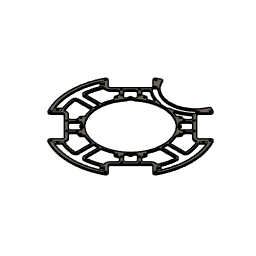
Frame_underside v16 (Autodesk Fusion 360 design; units mm, degrees)
Autodesk Fusion 360 part; units mm, degrees
note: some values were not read from the file. Set by a fixed rule: which face or edge a step refers to.
(part 1 of 3)
sketch "スケッチ1" plane through (0, 0, 0) normal (0, 0, 1) x (1, 0, 0)
  circle A0 centre (0, 0) radius 108
  circle A1 centre (0, 115.48) radius 45
  line L0 (0, 0) -> (76.3675, 76.3675)
  line L1 (0, 0) -> (108, 0) construction
  line L2 (0, 0) -> (76.3675, -76.3675)
  line L3 (76.3675, 76.3675) -> (58.5484, 58.5484)
  line L4 (76.3675, 76.3675) -> (96.1665, 56.5685)
  line L5 (76.3675, 76.3675) -> (56.5685, 96.1665)
  line L6 (96.1665, 56.5685) -> (78.3474, 38.7495)
  line L7 (78.3474, 38.7495) -> (58.5484, 58.5484)
  line L8 (56.5685, 96.1665) -> (38.7495, 78.3474)
  line L9 (38.7495, 78.3474) -> (58.5484, 58.5484)
  line L10 (56.5685, -96.1665) -> (38.7495, -78.3474)
  line L11 (38.7495, -78.3474) -> (58.5484, -58.5484)
  line L12 (78.3474, -38.7495) -> (58.5484, -58.5484)
  line L13 (96.1665, -56.5685) -> (78.3474, -38.7495)
  line L14 (76.3675, -76.3675) -> (96.1665, -56.5685)
  line L15 (76.3675, -76.3675) -> (56.5685, -96.1665)
  line L16 (0, 2.5) -> (0, 20)
  line L17 (-56.5685, -96.1665) -> (-38.7495, -78.3474)
  line L18 (-38.7495, -78.3474) -> (-58.5484, -58.5484)
  line L19 (-78.3474, -38.7495) -> (-58.5484, -58.5484)
  line L20 (-96.1665, -56.5685) -> (-78.3474, -38.7495)
  line L21 (-76.3675, -76.3675) -> (-96.1665, -56.5685)
  line L22 (-76.3675, -76.3675) -> (-56.5685, -96.1665)
  line L23 (0, 0) -> (-76.3675, -76.3675)
  line L24 (0, 0) -> (-76.3675, 76.3675)
  line L25 (-38.7495, 78.3474) -> (-58.5484, 58.5484)
  line L26 (-78.3474, 38.7495) -> (-58.5484, 58.5484)
  line L27 (-56.5685, 96.1665) -> (-38.7495, 78.3474)
  line L28 (-76.3675, 76.3675) -> (-56.5685, 96.1665)
  line L29 (-76.3675, 76.3675) -> (-96.1665, 56.5685)
  line L30 (-96.1665, 56.5685) -> (-78.3474, 38.7495)
  line L31 (-96.1665, 56.5685) -> (-99.7021, 53.033)
  line L32 (-99.7021, 53.033) -> (-78.3474, 31.6784)
  line L33 (-78.3474, 31.6784) -> (-31.6784, 78.3474)
  line L34 (-31.6784, 78.3474) -> (-53.033, 99.7021)
  line L35 (-53.033, 99.7021) -> (-56.5685, 96.1665)
  line L36 (-99.7021, -53.033) -> (-78.3474, -31.6784)
  line L37 (-78.3474, -31.6784) -> (-31.6784, -78.3474)
  line L38 (-31.6784, -78.3474) -> (-53.033, -99.7021)
  line L39 (-96.1665, -56.5685) -> (-99.7021, -53.033)
  line L40 (-53.033, -99.7021) -> (-56.5685, -96.1665)
  line L41 (96.1665, -56.5685) -> (99.7021, -53.033)
  line L42 (99.7021, -53.033) -> (78.3474, -31.6784)
  line L43 (78.3474, -31.6784) -> (31.6784, -78.3474)
  line L44 (31.6784, -78.3474) -> (53.033, -99.7021)
  line L45 (53.033, -99.7021) -> (56.5685, -96.1665)
  line L46 (96.1665, 56.5685) -> (99.7021, 53.033)
  line L47 (99.7021, 53.033) -> (78.3474, 31.6784)
  line L48 (78.3474, 31.6784) -> (31.6784, 78.3474)
  line L49 (31.6784, 78.3474) -> (53.033, 99.7021)
  line L50 (53.033, 99.7021) -> (56.5685, 96.1665)
  line L51 (-108, 0) -> (-103, 0)
  circle A2 centre (0, 0) radius 103
  line L52 (-103, 0) -> (-93, 0)
  circle A3 centre (0, 0) radius 93
  line L53 (0, 115.48) -> (0, 70.48)
  line L54 (0, 70.48) -> (0, 68.48)
  line L55 (0, 68.48) -> (0, 60.48)
  circle A4 centre (0, 115.48) radius 47
  circle A5 centre (0, 115.48) radius 55
  line L56 (0, 60.48) -> (0, 58.48)
  circle A6 centre (0, 115.48) radius 57
  line L57 (-93, 0) -> (-90, 0)
  circle A7 centre (0, 0) radius 90
  line L58 (0, 60.48) -> (0, 57.48)
  circle A8 centre (0, 0) radius 57.48
  circle A9 centre (0, 0) radius 60.48
  circle A10 centre (-42.7658, 42.7658) radius 3
  circle A11 centre (-42.7658, 42.7658) radius 1.45
  line L59 (-42.7658, 42.7658) -> (-44.8871, 40.6445)
  line L60 (-44.8871, 40.6445) -> (-42.1834, 37.9407)
  line L61 (-42.1834, 37.9407) -> (-37.9407, 42.1834)
  line L62 (-37.9407, 42.1834) -> (-42.7658, 42.7658)
  line L63 (-42.7658, 42.7658) -> (-40.6445, 44.8871)
  line L64 (-40.6445, 44.8871) -> (-37.9407, 42.1834)
  circle A12 centre (-42.7658, -42.7658) radius 3
  circle A13 centre (-42.7658, -42.7658) radius 1.45
  line L65 (-40.6445, -44.8871) -> (-37.9407, -42.1834)
  line L66 (-37.9407, -42.1834) -> (-42.1834, -37.9407)
  line L67 (-44.8871, -40.6445) -> (-42.1834, -37.9407)
  line L68 (-42.7658, -42.7658) -> (-44.8871, -40.6445)
  line L69 (-42.7658, -42.7658) -> (-40.6445, -44.8871)
  circle A14 centre (42.7658, -42.7658) radius 3
  circle A15 centre (42.7658, -42.7658) radius 1.45
  line L70 (44.8871, -40.6445) -> (42.1834, -37.9407)
  line L71 (42.1834, -37.9407) -> (37.9407, -42.1834)
  line L72 (40.6445, -44.8871) -> (37.9407, -42.1834)
  line L73 (42.7658, -42.7658) -> (40.6445, -44.8871)
  line L74 (42.7658, -42.7658) -> (44.8871, -40.6445)
  circle A16 centre (42.7658, 42.7658) radius 3
  circle A17 centre (42.7658, 42.7658) radius 1.45
  line L75 (40.6445, 44.8871) -> (37.9407, 42.1834)
  line L76 (37.9407, 42.1834) -> (42.1834, 37.9407)
  line L77 (44.8871, 40.6445) -> (42.1834, 37.9407)
  line L78 (42.7658, 42.7658) -> (44.8871, 40.6445)
  line L79 (42.7658, 42.7658) -> (40.6445, 44.8871)
  line L80 (-103, 0) -> (-103, 5)
  line L81 (-103, 5) -> (-57.2621, 5)
  line L82 (-103, 0) -> (-103, -5)
  line L83 (-103, -5) -> (-57.2621, -5)
  line L84 (-103, 5) -> (-103, 8)
  line L85 (-103, 8) -> (-56.9206, 8)
  line L86 (-103, -5) -> (-103, -8)
  line L87 (-103, -8) -> (-56.9206, -8)
  line L88 (103, 8) -> (56.9206, 8)
  line L89 (103, 5) -> (57.2621, 5)
  line L90 (103, -5) -> (57.2621, -5)
  line L91 (103, -8) -> (56.9206, -8)
  line L92 (0, -108) -> (5, -108)
  line L93 (5, -108) -> (0, -108)
  line L94 (0, -108) -> (0, -57.4798)
  line L95 (0, -57.4798) -> (5, -57.4798)
  line L96 (5, -57.4798) -> (5, -108)
  line L97 (0, -108) -> (-5, -108)
  line L98 (-5, -108) -> (-5, -57.4798)
  line L99 (-5, -57.4798) -> (0, -57.4798)
  line L100 (0, -57.4798) -> (0, -108)
  line L101 (-5, -57.4798) -> (-8, -57.4798)
  line L102 (-8, -57.4798) -> (-8, -108)
  line L103 (-8, -108) -> (-5, -108)
  line L104 (-5, -108) -> (-5, -57.4798)
  line L105 (5, -108) -> (8, -108)
  line L106 (8, -108) -> (8, -57.4798)
  line L107 (8, -57.4798) -> (5, -57.4798)
  line L108 (5, -57.4798) -> (5, -108)
  line L109 (0, -108) -> (0, -104.5)
  circle A18 centre (0, 0) radius 104.5
  line L110 (-31.6784, -78.3474) -> (-32.739, -77.2868)
  line L111 (-32.739, -77.2868) -> (-50.7732, -95.3209)
  circle A19 centre (-48.1818, -92.7295) radius 1.65
  line L112 (-78.3474, -31.6784) -> (-77.2868, -32.739)
  line L113 (-77.2868, -32.739) -> (-98.6414, -54.0937)
  circle A20 centre (-92.7295, -48.1818) radius 1.65
  line L114 (31.6784, -78.3474) -> (32.739, -77.2868)
  line L115 (32.739, -77.2868) -> (54.0937, -98.6414)
  circle A21 centre (48.1818, -92.7295) radius 1.65
  line L116 (78.3474, -31.6784) -> (77.2868, -32.739)
  line L117 (77.2868, -32.739) -> (98.6414, -54.0937)
  circle A22 centre (92.7295, -48.1818) radius 1.65
  line L118 (-99.7021, 53.033) -> (-98.6414, 54.0937)
  line L119 (-98.6414, 54.0937) -> (-77.2868, 32.739)
  circle A23 centre (-92.7295, 48.1818) radius 1.65
  circle A24 centre (92.7295, -48.1818) radius 1.65
  circle A25 centre (48.1818, 92.7295) radius 1.65
  circle A26 centre (-92.7295, 48.1818) radius 1.65
  line L120 (31.6784, 78.3474) -> (32.739, 77.2868)
  line L121 (32.739, 77.2868) -> (54.0937, 98.6414)
  circle A27 centre (48.1818, -92.7295) radius 1.65
  circle A28 centre (92.7295, 48.1818) radius 1.65
  circle A29 centre (-48.1818, 92.7295) radius 1.65
  line L122 (-58.5484, 58.5484) -> (-66.4857, 50.6112)
  line L123 (-66.4857, 50.6112) -> (-50.6112, 66.4857)
  line L124 (-50.6112, 66.4857) -> (-29.0444, 44.919)
  line L125 (-29.0444, 44.919) -> (-44.919, 29.0444)
  line L126 (-44.919, 29.0444) -> (-66.4857, 50.6112)
  line L127 (-66.4857, 50.6112) -> (-64.7179, 52.3789)
  line L128 (-64.7179, 52.3789) -> (-43.1512, 30.8122)
  line L129 (-66.4857, 50.6112) -> (-68.2535, 48.8434)
  line L130 (-68.2535, 48.8434) -> (-46.6867, 27.2766)
  line L131 (-46.6867, 27.2766) -> (-44.919, 29.0444)
  line L132 (-48.8434, 68.2535) -> (-27.2766, 46.6867)
  line L133 (-52.3789, 64.7179) -> (-30.8122, 43.1512)
  line L134 (-29.0444, 44.919) -> (-27.2766, 46.6867)
  line L135 (-66.4857, 50.6112) -> (-64.0816, 48.207)
  circle A30 centre (-64.0816, 48.207) radius 1.65
  circle A31 centre (-48.207, 64.0816) radius 1.65
  line L136 (-64.0816, 48.207) -> (-55.172, 39.2975)
  line L137 (-55.172, 39.2975) -> (-39.2975, 55.172)
  circle A32 centre (-55.172, 39.2975) radius 1.65
  circle A33 centre (-39.2975, 55.172) radius 1.65
  circle A34 centre (-48.207, -64.0816) radius 1.65
  circle A35 centre (-39.2975, -55.172) radius 1.65
  circle A36 centre (-64.0816, -48.207) radius 1.65
  circle A37 centre (-55.172, -39.2975) radius 1.65
  line L138 (-64.7179, -52.3789) -> (-43.1512, -30.8122)
  line L139 (-68.2535, -48.8434) -> (-46.6867, -27.2766)
  line L140 (-44.919, -29.0444) -> (-46.6867, -27.2766)
  line L141 (-27.2766, -46.6867) -> (-29.0444, -44.919)
  line L142 (-48.8434, -68.2535) -> (-27.2766, -46.6867)
  line L143 (-29.0444, -44.919) -> (-50.6112, -66.4857)
  line L144 (-52.3789, -64.7179) -> (-30.8122, -43.1512)
  line L145 (-44.919, -29.0444) -> (-29.0444, -44.919)
  line L146 (-66.4857, -50.6112) -> (-44.919, -29.0444)
  circle A38 centre (64.0816, -48.207) radius 1.65
  circle A39 centre (55.172, -39.2975) radius 1.65
  circle A40 centre (48.207, -64.0816) radius 1.65
  circle A41 centre (39.2975, -55.172) radius 1.65
  line L147 (52.3789, -64.7179) -> (30.8122, -43.1512)
  line L148 (48.8434, -68.2535) -> (27.2766, -46.6867)
  line L149 (29.0444, -44.919) -> (27.2766, -46.6867)
  line L150 (46.6867, -27.2766) -> (44.919, -29.0444)
  line L151 (68.2535, -48.8434) -> (46.6867, -27.2766)
  line L152 (44.919, -29.0444) -> (66.4857, -50.6112)
  line L153 (64.7179, -52.3789) -> (43.1512, -30.8122)
  line L154 (29.0444, -44.919) -> (44.919, -29.0444)
  line L155 (50.6112, -66.4857) -> (29.0444, -44.919)
  circle A42 centre (48.207, 64.0816) radius 1.65
  circle A43 centre (39.2975, 55.172) radius 1.65
  circle A44 centre (64.0816, 48.207) radius 1.65
  circle A45 centre (55.172, 39.2975) radius 1.65
  line L156 (64.7179, 52.3789) -> (43.1512, 30.8122)
  line L157 (68.2535, 48.8434) -> (46.6867, 27.2766)
  line L158 (44.919, 29.0444) -> (46.6867, 27.2766)
  line L159 (27.2766, 46.6867) -> (29.0444, 44.919)
  line L160 (48.8434, 68.2535) -> (27.2766, 46.6867)
  line L161 (29.0444, 44.919) -> (50.6112, 66.4857)
  line L162 (52.3789, 64.7179) -> (30.8122, 43.1512)
  line L163 (44.919, 29.0444) -> (29.0444, 44.919)
  line L164 (66.4857, 50.6112) -> (44.919, 29.0444)
  line L165 (-60.273, 5) -> (-60.273, -5)
  line L166 (-31.6784, 78.3474) -> (-28.9756, 81.0502)
  line L167 (31.6784, 78.3474) -> (28.9756, 81.0502)
  line L168 (60.273, -5) -> (60.273, 5)
  line L169 (-5, -60.273) -> (5, -60.273)
  line L170 (-38.7495, 78.3474) -> (-34.0326, 83.0643)
  line L171 (38.7495, 78.3474) -> (32.618, 84.4789)
  line L172 (38.7495, 78.3474) -> (38.0423, 77.6403)
  line L173 (38.0423, 77.6403) -> (31.921, 83.7617)
  line L174 (-38.7495, 78.3474) -> (-38.0423, 77.6403)
  line L175 (-38.0423, 77.6403) -> (-33.3352, 82.3475)
  line L176 (-38.0423, 77.6403) -> (-40.4063, 75.2764)
  line L177 (38.0423, 77.6403) -> (40.4063, 75.2764)
  dimension "d1" = 216
  dimension "d2" = 90
  dimension "d4" = 45
  dimension "d5" = 25.2
  dimension "d6" = 28
  dimension "d7" = 28
  dimension "d9" = 25.2
  dimension "d10" = 28
  dimension "d11" = 25.2
  dimension "d12" = 28
  dimension "d13" = 5
  dimension "d14" = 30.2
  dimension "d15" = 66
  dimension "d16" = 30.2
  dimension "d17" = 5
  dimension "d18" = 10
  dimension "d20" = 2
  dimension "d21" = 8
  dimension "d22" = 2
  dimension "d23" = 3
  dimension "d24" = 3
  dimension "d25" = 2.9
  dimension "d26" = 6
  dimension "d27" = 3
  dimension "d29" = 360
  dimension "d30" = 5
  dimension "d31" = 5
  dimension "d32" = 3
  dimension "d33" = 3
  dimension "d34" = 5
  dimension "d35" = 5
  dimension "d36" = 5
  dimension "d37" = 3
  dimension "d38" = 3
  dimension "d39" = 3.5
  dimension "d40" = 1.5
  dimension "d42" = 3.3
  dimension "d43" = 1.5
  dimension "d45" = 3.3
  dimension "d46" = 1.5
  dimension "d48" = 3.3
  dimension "d49" = 1.5
  dimension "d51" = 3.3
  dimension "d52" = 1.5
  dimension "d54" = 3.3
  dimension "d56" = 360
  dimension "d57" = 1.5
  dimension "d59" = 360
  dimension "d60" = 11.225
  dimension "d61" = 22.45
  dimension "d62" = 30.5
  dimension "d63" = 22.45
  dimension "d64" = 2.5
  dimension "d65" = 2.5
  dimension "d66" = 30.5
  dimension "d67" = 3.4
  dimension "d68" = 3.3
  dimension "d69" = 12.6
  dimension "d70" = 22.45
  dimension "d71" = 3.3
  dimension "d72" = 3.3
  dimension "d74" = 360
  dimension "d77" = 1
  constraint coincident A0.centre L0.start
  constraint horizontal L1
  constraint coincident A0 L0.end
  constraint coincident A0 L2.end
  constraint perpendicular L0 L2
  constraint perpendicular L2 L3
  constraint perpendicular L3 L4
  constraint perpendicular L0 L5
  constraint perpendicular L4 L6
  constraint perpendicular L6 L7
  constraint perpendicular L5 L8
  constraint perpendicular L8 L9
  constraint symmetric L0.end L1 L2.end
  constraint symmetric L1 L4.end L13.start
  constraint symmetric L1 L5.end L10.start
  constraint symmetric L1 L6.end L12.start
  constraint symmetric L1 L3.end L11.end
  constraint symmetric L1 L8.end L10.end
  constraint symmetric A0.centre L16 L0.start
  constraint symmetric L0.end L16 L24.end
  constraint symmetric L2.end L16 L21.start
  constraint symmetric L4.end L16 L29.end
  constraint symmetric L5.end L16 L27.start
  constraint symmetric L6.end L16 L26.start
  constraint symmetric L3.end L16 L25.end
  constraint symmetric L8.end L16 L25.start
  constraint symmetric L10.start L16 L17.start
  constraint symmetric L10.end L16 L17.end
  constraint symmetric L11.end L16 L18.end
  constraint symmetric L12.start L16 L19.start
  constraint symmetric L13.start L16 L20.start
  constraint perpendicular L30 L31
  constraint perpendicular L26 L32
  constraint perpendicular L32 L33
  constraint perpendicular L33 L34
  constraint symmetric L1 L27.start L17.start
  constraint symmetric L1 L29.end L20.start
  constraint symmetric L1 L31.end L36.start
  constraint symmetric L1 L32.end L36.end
  constraint symmetric L1 L33.end L37.end
  constraint symmetric L1 L34.end L38.end
  constraint symmetric L16 L27.start L5.end
  constraint symmetric L16 L29.end L4.end
  constraint symmetric L16 L31.end L46.end
  constraint symmetric L16 L32.end L47.end
  constraint symmetric L16 L33.end L48.end
  constraint symmetric L16 L34.end L49.end
  constraint symmetric L16 L36.start L41.end
  constraint symmetric L16 L36.end L42.end
  constraint symmetric L16 L37.end L43.end
  constraint symmetric L16 L38.end L44.end
  constraint symmetric L16 L20.start L13.start
  constraint symmetric L16 L17.start L10.start
  constraint coincident A0 L51.start
  constraint horizontal L51
  constraint coincident L51.end A2
  constraint parallel L51 L52
  constraint coincident L52.end A3
  constraint coincident A1.centre L53.start
  constraint coincident A1 L53.end
  constraint vertical L53
  constraint parallel L53 L54
  constraint parallel L53 L55
  constraint concentric A1 A4
  constraint coincident L54.end A4
  constraint concentric A1 A5
  constraint coincident L55.end A5
  constraint parallel L55 L56
  constraint concentric A4 A6
  constraint coincident L56.end A6
  constraint concentric A2 A7
  constraint coincident L57.end A7
  constraint parallel L56 L58
  constraint concentric A7 A8
  constraint coincident L58.end A8
  constraint concentric A3 A9
  constraint coincident L55.end A9
  constraint tangent A5 A9
  constraint coincident A9 A10.centre
  constraint coincident L24 A10.centre
  constraint tangent A8 A10
  constraint concentric A10 A11
  constraint coincident A10.centre A11.centre
  constraint coincident A10 L59.end
  constraint tangent A9 L59
  constraint perpendicular L24 L59
  constraint tangent A10 L60
  constraint perpendicular L24 L61
  constraint tangent A9 L63
  constraint perpendicular L52 L80
  constraint coincident A8 L81.end
  constraint perpendicular L80 L81
  constraint perpendicular L52 L82
  constraint coincident A8 L83.end
  constraint perpendicular L82 L83
  constraint perpendicular L81 L84
  constraint coincident A8 L85.end
  constraint perpendicular L84 L85
  constraint perpendicular L83 L86
  constraint coincident A8 L87.end
  constraint perpendicular L86 L87
  constraint symmetric L16 L80.end L89.start
  constraint symmetric L16 L81.end L89.end
  constraint symmetric L16 L82.end L90.start
  constraint symmetric L16 L83.end L90.end
  constraint symmetric L16 L84.end L88.start
  constraint symmetric L16 L85.end L88.end
  constraint symmetric L16 L86.end L91.start
  constraint symmetric L16 L87.end L91.end
  constraint coincident A0 L92.start
  constraint horizontal L92
  constraint horizontal L93
  constraint vertical L94
  constraint horizontal L95
  constraint vertical L96
  constraint horizontal L97
  constraint vertical L98
  constraint horizontal L99
  constraint vertical L100
  constraint horizontal L101
  constraint vertical L102
  constraint horizontal L103
  constraint vertical L104
  constraint horizontal L105
  constraint vertical L106
  constraint horizontal L107
  constraint vertical L108
  constraint perpendicular L97 L109
  constraint concentric A3 A18
  constraint coincident L109.end A18
  constraint coincident L37 L110.end
  constraint coincident A0 L111.end
  constraint perpendicular L110 L111
  constraint perpendicular L36 L112
  constraint coincident L39 L113.end
  constraint perpendicular L39 L113
  constraint perpendicular L44 L114
  constraint coincident L45 L115.end
  constraint perpendicular L45 L115
  constraint perpendicular L42 L116
  constraint coincident L41 L117.end
  constraint perpendicular L41 L117
  constraint perpendicular L32 L118
  constraint coincident L33 L119.end
  constraint perpendicular L33 L119
  constraint perpendicular L49 L120
  constraint coincident L50 L121.end
  constraint perpendicular L50 L121
  constraint perpendicular L24 L122
  constraint parallel L25 L123
  constraint perpendicular L33 L124
  constraint perpendicular L124 L125
  constraint perpendicular L126 L127
  constraint coincident L125 L128.end
  constraint perpendicular L125 L128
  constraint perpendicular L126 L129
  constraint perpendicular L26 L130
  constraint symmetric L24 L127.end L133.start
  constraint symmetric L24 L128.end L133.end
  constraint symmetric L24 L129.end L132.start
  constraint symmetric L24 L130.end L132.end
  constraint perpendicular L122 L135
  constraint coincident L135.end A30.centre
  constraint symmetric L24 A30 A31
  constraint perpendicular L33 L136
  constraint perpendicular L126 L137
  constraint coincident L136.end L137.start
  constraint coincident L137.end A33.centre
  constraint coincident A9 L165.start
  constraint coincident L81 L165.start
  constraint coincident A9 L165.end
  constraint coincident L83 L165.end
  constraint perpendicular L83 L165
  constraint coincident A1 L166.end
  constraint perpendicular L34 L166
  constraint coincident A1 L167.end
  constraint perpendicular L49 L167
  constraint coincident A9 L168.start
  constraint coincident L90 L168.start
  constraint coincident A9 L168.end
  constraint coincident L89 L168.end
  constraint perpendicular L89 L168
  constraint coincident L104 L169.start
  constraint coincident A9 L169.start
  constraint coincident L108 L169.end
  constraint coincident A9 L169.end
  constraint perpendicular L108 L169
  constraint coincident A4 L170.end
  constraint perpendicular L34 L170
  constraint coincident A1 L171.end
  constraint perpendicular L170 L171
  constraint perpendicular L9 L172
  constraint coincident A1 L173.end
  constraint perpendicular L172 L173
  constraint perpendicular L25 L174
  constraint coincident A4 L175.end
  constraint perpendicular L174 L175
  constraint coincident A6 L176.end
  constraint perpendicular L174 L176
  constraint coincident A6 L177.end
  constraint perpendicular L176 L177
  measures "d1" diameter of A0
  measures "d2" diameter of A1
  measures "d4" angle of L0 L1
  measures "d5" distance of L0.end L3.end
  measures "d6" distance of L0.end L4.end
  measures "d7" distance of L0.end L5.end
  measures "d9" distance of L4.end L6.end
  measures "d10" distance of L6.end L3.end
  measures "d11" distance of L5.end L8.end
  measures "d12" distance of L8.end L3.end
  measures "d13" distance of L29.end L31.end
  measures "d14" distance of L31.end L32.end
  measures "d15" distance of L32.end L33.end
  measures "d16" distance of L33.end L34.end
  measures "d17" distance of L51.start L51.end
  measures "d18" distance of L51.end L52.end
  measures "d20" distance of L53.end L54.end
  measures "d21" distance of L54.end L55.end
  measures "d22" distance of L55.end L56.end
  measures "d23" distance of L52.end L57.end
  measures "d24" distance of L55.end L58.end
  measures "d25" diameter of A11
  measures "d26" distance of L60.end L61.end
  measures "d27" distance of A10.centre L63.end
  measures "d30" distance of L51.end L80.end
  measures "d31" distance of L51.end L82.end
  measures "d32" distance of L80.end L84.end
  measures "d33" distance of L82.end L86.end
  measures "d34" distance of L92.start L92.end
  measures "d35" distance of L92.end L92.start
  measures "d36" distance of L92.start L97.end
  measures "d37" distance of L98.end L101.end
  measures "d38" distance of L92.end L105.end
  measures "d39" distance of L92.start L109.end
  measures "d40" distance of L37.end L110.end
  measures "d42" diameter of A19
  measures "d43" distance of L36.end L112.end
  measures "d45" diameter of A20
  measures "d46" distance of L43.end L114.end
  measures "d48" diameter of A21
  measures "d49" distance of L42.end L116.end
  measures "d51" diameter of A22
  measures "d52" distance of L31.end L118.end
  measures "d54" diameter of A23
  measures "d57" distance of L48.end L120.end
  measures "d60" distance of L25.end L122.end
  measures "d61" distance of L122.end L123.end
  measures "d62" distance of L123.end L124.end
  measures "d63" distance of L124.end L125.end
  measures "d64" distance of L122.end L127.end
  measures "d65" distance of L122.end L129.end
  measures "d66" distance of L129.end L130.end
  measures "d67" distance of L122.end L135.end
  measures "d68" diameter of A30
  measures "d69" distance of L135.end L136.end
  measures "d70" distance of L136.end L137.end
  measures "d71" diameter of A32
  measures "d72" diameter of A33
  measures "d77" distance of L8.end L172.end
extrude "押し出し1" add sketch "スケッチ1" along normal blind 2 contours A0 L42 L47 A18 A22 A24 A28 | A0 L6 L47 A18 A28 | A0 L42 L117 A22 A24 | A0 L13 A18 L117 A22 A24 | L6 A2 A18 A28 | L42 L47 A2 A18 A22 A24 A28 | A0 L8 A6 | L6 L47 A2 A3 A28 | L47 A2 A28 | L13 A2 A18 A22 A24 | L42 A2 A22 A24 | A0 L8 A5 A6 A18 | L6 L47 A3 A7 | A0 L10 A18 L115 A21 A27 | L13 A2 A3 L117 A22 A24 | L42 A2 A3 L117 A22 A24 | A0 A5 A18 A25 L121 | L8 A2 A5 A18 | L6 L7 L47 L48 A7 L157 | L47 A3 A7 L88 | A0 L44 L115 A21 A27 | L10 A2 A18 A21 A27 | L13 A3 A7 L117 | L42 A3 A7 L117 | L42 A3 A7 L91 | A0 L49 A25 L121 | A2 A5 A18 A25 | L8 A2 A5 | A3 A7 L88 L89 | A0 L44 L106 A18 A21 A27 | L10 A2 A3 L115 A21 A27 | L12 L13 L43 A7 L117 L151 | L42 L43 A7 L116 L117 | A3 A7 L90 L91 | A0 L49 A4 A18 A25 | L8 A2 A3 A5 A25 L121 | L0 L7 L48 L156 | L0 L9 L48 L162 | A0 L27 A6 | A0 L27 A5 A6 A18 | L7 L48 A44 L157 L164 | A7 A9 L88 L89 | A0 L96 L106 L108 A18 | L10 A3 A7 L115 | A7 A9 L90 L91 | A0 A1 A4 A18 | L8 A3 A7 L121 | L7 L48 A44 L156 L164 | L9 L48 A42 L161 L162 | L9 A5 A6 L177 | L9 L48 A6 L160 | A0 L34 A5 A18 A29 | L48 A9 A44 A45 L157 L164 | A8 A9 L88 L157 | A8 A9 L88 L89 | A0 L94 L96 L100 L108 L109 A18 | A2 L96 L106 L108 A18 | L44 A2 L106 A18 A21 A27 | L10 L11 L43 A7 L115 L148 | L44 A2 A3 L115 A21 A27 | L44 A3 A7 L115 | L2 L11 L43 L147 | L2 L12 L43 L153 | L12 L43 A38 L151 L152 | A8 A9 L90 L91 | A8 A9 L91 L151 | L49 A2 A4 A18 A25 | A1 A2 A4 A18 | L49 A2 A3 A25 L121 | L8 A7 L121 L171 | L49 A3 A7 L121 | L0 A16 A17 L78 | L0 A16 A17 L79 | L48 A9 A44 A45 L156 L164 | L48 A9 A42 A43 L161 L162 | L9 L48 A42 L160 L161 | L9 A5 L172 L177 | L48 A5 A6 L177 | A0 L34 A4 A18 A29 | A0 L30 A18 L119 A23 A26 | A2 A5 A18 A29 | L27 A2 A5 A18 | A8 A9 L157 L164 | A8 L89 L90 L168 | A0 L94 L98 L100 L104 L109 A18 | A2 L94 L96 L100 L108 A18 | L44 A2 A21 A27 | L43 L44 A7 L114 L115 | L44 A3 A7 L106 | L11 L43 A40 L147 L155 | L12 L43 A38 L152 L153 | L43 A9 A38 A39 L151 L152 | A8 A9 L151 L152 | A1 A2 A3 A4 | L49 A2 A3 A4 | A0 A1 A4 A18 | L49 A2 A25 | L121 L171 L172 L173 | L49 A7 L121 L171 | L49 A3 A4 A7 | A9 A16 A17 L75 L79 | A8 A9 L77 L156 | A8 A9 L156 L164 | A8 A9 L161 L162 | A8 A9 L75 L162 | L48 A9 A42 A43 L160 L161 | L48 A5 A6 A9 | A0 L32 L119 A23 A26 | L30 A2 A18 A23 A26 | L27 A2 A5 | L27 L34 A2 A3 A5 A29 | A0 L98 L102 L104 A18 | A2 L94 L98 L100 L104 A18 | A3 A7 L96 L106 L108 | L11 L43 A40 L148 L155 | L2 A14 A15 L73 | L2 A14 A15 L74 | L43 A9 A38 A39 L152 L153 | L43 A9 A40 A41 L147 L155 | A8 A9 L152 L153 | A1 A3 A4 A7 L171 | A1 A2 A4 A18 | L34 A2 A4 A18 A29 | L49 L121 L171 L173 | L49 A4 A7 L171 | A9 A16 A17 L77 L78 | L0 A9 A16 A17 | A8 A16 L75 | L0 A9 A16 A17 | A8 A16 L77 | A8 A9 L160 L161 | A6 L58 A8 A9 L160 | L56 A6 L58 A9 | A0 L32 L51 A18 A23 A26 | L30 A2 A3 L119 A23 A26 | A0 L38 L102 A18 A19 | A2 L98 L102 L104 A18 | A7 A9 L96 L106 L108 | L43 A9 A40 A41 L148 L155 | A9 A14 A15 L72 L73 | A8 A9 L70 L153 | A8 A9 L72 L147 | A8 A9 L147 L155 | A4 A7 L171 | L34 A2 A3 A4 | A1 A2 A3 A4 | L49 A4 L171 L173 | L33 A5 A6 A9 | L56 A6 L58 A9 | A6 L58 A8 A9 L132 | L34 A2 A29 | A0 L36 L51 A18 A20 | L30 A3 A7 L119 | L27 L34 A3 A7 | A0 L38 L111 A19 | L38 A2 L102 A18 A19 | A8 A9 L95 L106 L107 L148 | A9 L96 L106 L107 L108 | A8 A9 L148 L155 | L2 A9 A14 A15 | A8 A14 L72 | A9 A14 A15 L70 L74 | L2 A9 A14 A15 | A8 A14 L70 | A1 A7 L171 | A1 A4 A7 L171 L173 | L34 A3 A4 A7 | A1 A3 A4 A7 | A1 L54 A4 L166 | A1 L54 A4 L167 | L33 A5 A6 L176 | A0 L36 L113 A20 | L32 L51 A2 L80 L84 L85 A18 A23 A26 | L36 L51 A2 L82 L86 L87 A18 A20 | L26 L30 L33 A7 L119 L130 | L32 A3 A7 L119 | L32 A2 A3 L119 A23 A26 | L24 L25 L33 L123 L133 | L24 L26 L33 L122 L123 L128 | L27 L34 A7 L170 | L25 L33 A6 L132 | L25 A5 A6 L176 | A0 L17 A18 L111 A19 | A3 A7 L98 L102 L104 | L94 L95 L96 L100 L108 L169 | A1 A4 L167 L173 | A1 A4 A7 L166 | L34 A4 A7 L170 | L25 A5 L174 L176 | A8 A9 L124 L132 | L33 A9 L124 L132 A31 A33 | A0 L20 A18 L113 A20 | A2 L80 L81 | A2 L82 L83 | L32 A2 A23 A26 | L32 L33 A7 L119 | L32 A3 A7 L85 | L25 L33 L123 L124 L133 A31 | L26 L33 L122 L123 L126 L127 L128 L135 A30 | L34 L170 L174 L175 | L25 L33 L124 L132 A31 | L38 A2 A3 L111 A19 | L38 A2 A19 | L38 A3 A7 L102 | A7 A9 L98 L102 L104 | L94 L98 L99 L100 L104 L169 | A8 A9 L99 L101 L102 L142 | L34 A4 L170 L175 | A8 A9 L124 L133 | A9 L124 L133 L137 A33 | A2 L81 L84 L85 | A2 L83 L86 L87 | L36 A2 A20 | L26 L33 L126 L129 L130 L135 A30 | A3 A7 L81 L85 | L33 L126 L128 A30 L136 L137 A32 | L33 L124 L133 A31 L137 A33 | L17 A2 A18 A19 | L38 A3 A7 L111 | A9 L98 L101 L102 L104 | A8 A9 L142 L143 | A8 A9 L64 L133 | L20 A2 A18 A20 | A3 A7 L83 L87 | L36 A2 A3 L113 A20 | L33 A9 L126 L130 A30 L136 A32 | A7 A9 L81 L85 | L24 A10 A11 L63 | L24 A10 A11 L59 | A9 L126 L128 L137 A32 | L17 A2 A3 L111 A19 | L37 L38 A7 L110 L111 | L17 A3 A7 L111 | A8 A9 L143 L144 | L37 A9 A34 A35 L142 L143 | L23 A9 A12 A13 | A8 A12 L67 | A8 A12 L65 | L23 A9 A12 A13 | A8 A9 L138 L146 | A8 A9 L67 L138 | A8 A9 L65 L144 | L24 A9 A10 A11 | A8 A10 L62 | A8 A10 L60 | L24 A10 A11 L62 | A8 A9 L60 L128 | A8 A9 L126 L128 | A9 A10 A11 L62 | A8 A10 L62 L64 | A9 A10 A11 L63 L64 | L20 A2 A3 L113 A20 | L36 A3 A7 L87 | A7 A9 L83 L87 | L36 A3 A7 L113 | A8 A9 L85 L130 | A8 A9 L126 L130 | A8 A9 L81 L85 | A9 A10 A11 L59 L60 | L17 L18 L37 A7 L111 L142 | L37 A9 A34 A35 L143 L144 | L18 L37 A34 L142 L143 | A9 A12 A13 L67 L68 | A8 A9 L139 L146 | L37 A9 A36 A37 L138 L146 | L20 A3 A7 L113 | A8 L81 L83 L165 | A8 A9 L83 L87 | L36 L37 A7 L112 L113 | A9 A12 A13 L65 L69 | L23 A12 A13 L68 | A8 A9 L87 L139 | L37 A9 A36 A37 L139 L146 | L19 L37 A36 L138 L146 | L19 L23 L37 L138 | L18 L23 L37 L144 | L18 L37 A34 L143 L144 | L19 L20 L37 A7 L113 L139 | L23 A12 A13 L69 | L19 L37 A36 L139 L146
sketch "スケッチ2" plane through (0, 0, 2) normal (0, 0, 1) x (-1, 0, 0)
  circle A0 centre (42.7658, -42.7658) radius 1.45
  circle A1 centre (-42.7658, 42.7658) radius 1.45
  line L0 (-48.488, 36.149) -> (-61.1824, 48.8434)
  line L1 (-61.1824, 48.8434) -> (-48.8434, 61.1824)
  line L2 (-48.8434, 61.1824) -> (-36.149, 48.488)
  arc A2 (-36.149, 48.488) -> (-40.5925, 44.8339) centre (0, 0) ccw
  arc A3 (-40.5925, 44.8339) -> (-44.8339, 40.5925) centre (-42.7658, 42.7658) ccw
  arc A4 (-44.8339, 40.5925) -> (-48.488, 36.149) centre (0, 0) ccw
  arc A5 (-82.5418, 35.8727) -> (-89.6437, 8) centre (0, 0) ccw
  line L3 (-82.5418, 35.8727) -> (-78.3474, 31.6784)
  line L4 (-78.3474, 31.6784) -> (-64.7179, 45.3079)
  line L5 (-64.7179, 45.3079) -> (-51.3551, 31.945)
  arc A6 (-51.3551, 31.945) -> (-59.9486, 8) centre (0, 0) ccw
  line L6 (-59.9486, 8) -> (-89.6437, 8)
  circle A7 centre (-64.0816, 48.207) radius 1.65
  line L7 (31.945, -51.3551) -> (45.3079, -64.7179)
  line L8 (45.3079, -64.7179) -> (37.4856, -72.5402)
  arc A8 (37.4856, -72.5402) -> (10.7877, -59.5101) centre (0, -115.48) ccw
  arc A9 (10.7877, -59.5101) -> (31.945, -51.3551) centre (0, 0) ccw
  arc A10 (-89.6437, -8) -> (-82.5418, -35.8727) centre (0, 0) ccw
  line L9 (-89.6437, -8) -> (-59.9486, -8)
  arc A11 (-59.9486, -8) -> (-51.3551, -31.945) centre (0, 0) ccw
  line L10 (-51.3551, -31.945) -> (-64.7179, -45.3079)
  line L11 (-64.7179, -45.3079) -> (-78.3474, -31.6784)
  line L12 (-78.3474, -31.6784) -> (-82.5418, -35.8727)
  circle A12 centre (-48.207, -64.0816) radius 1.65
  circle A13 centre (42.7658, 42.7658) radius 1.45
  line L13 (-45.3079, -64.7179) -> (-31.945, -51.3551)
  arc A14 (-31.945, -51.3551) -> (-10.7877, -59.5101) centre (0, 0) ccw
  arc A15 (-10.7877, -59.5101) -> (-37.4856, -72.5402) centre (0, -115.48) ccw
  line L14 (-37.4856, -72.5402) -> (-45.3079, -64.7179)
  circle A16 centre (-55.172, 39.2975) radius 1.65
  circle A17 centre (-92.7295, -48.1818) radius 1.65
  circle A18 centre (-92.7295, 48.1818) radius 1.65
  circle A19 centre (39.2975, -55.172) radius 1.65
  arc A20 (-92.3273, 45.6582) -> (-92.3273, -45.6582) centre (0, 0) ccw
  line L15 (-92.3273, 45.6582) -> (-84.8162, 38.1472)
  arc A21 (-84.8162, 38.1472) -> (-92.8655, 5) centre (0, 0) ccw
  line L16 (-92.8655, 5) -> (-60.273, 5)
  line L17 (-60.273, 5) -> (-60.273, -5)
  line L18 (-60.273, -5) -> (-92.8655, -5)
  arc A22 (-92.8655, -5) -> (-84.8162, -38.1472) centre (0, 0) ccw
  line L19 (-84.8162, -38.1472) -> (-92.3273, -45.6582)
  circle A23 centre (48.207, -64.0816) radius 1.65
  circle A24 centre (-39.2975, -55.172) radius 1.65
  circle A25 centre (-42.7658, -42.7658) radius 1.45
  circle A26 centre (92.7295, 48.1818) radius 1.65
  circle A27 centre (92.7295, -48.1818) radius 1.65
  circle A28 centre (48.207, 64.0816) radius 1.65
  arc A29 (82.5418, -35.8727) -> (89.6437, -8) centre (0, 0) ccw
  line L20 (82.5418, -35.8727) -> (78.3474, -31.6784)
  line L21 (78.3474, -31.6784) -> (64.7179, -45.3079)
  line L22 (64.7179, -45.3079) -> (51.3551, -31.945)
  arc A30 (51.3551, -31.945) -> (59.9486, -8) centre (0, 0) ccw
  line L23 (59.9486, -8) -> (89.6437, -8)
  circle A31 centre (39.2975, 55.172) radius 1.65
  circle A32 centre (-48.207, 64.0816) radius 1.65
  arc A33 (92.3273, -45.6582) -> (92.3273, 45.6582) centre (0, 0) ccw
  line L24 (92.3273, -45.6582) -> (84.8162, -38.1472)
  arc A34 (84.8162, -38.1472) -> (92.8655, -5) centre (0, 0) ccw
  line L25 (92.8655, -5) -> (60.273, -5)
  line L26 (60.273, -5) -> (60.273, 5)
  line L27 (60.273, 5) -> (92.8655, 5)
  arc A35 (92.8655, 5) -> (84.8162, 38.1472) centre (0, 0) ccw
  line L28 (84.8162, 38.1472) -> (92.3273, 45.6582)
  line L29 (48.488, -36.149) -> (61.1824, -48.8434)
  line L30 (61.1824, -48.8434) -> (48.8434, -61.1824)
  line L31 (48.8434, -61.1824) -> (36.149, -48.488)
  arc A36 (36.149, -48.488) -> (40.5925, -44.8339) centre (0, 0) ccw
  arc A37 (40.5925, -44.8339) -> (44.8339, -40.5925) centre (42.7658, -42.7658) ccw
  arc A38 (44.8339, -40.5925) -> (48.488, -36.149) centre (0, 0) ccw
  circle A39 centre (64.0816, -48.207) radius 1.65
  circle A40 centre (55.172, -39.2975) radius 1.65
  circle A41 centre (48.1818, -92.7295) radius 1.65
  line L32 (-61.1824, -48.8434) -> (-48.488, -36.149)
  arc A42 (-48.488, -36.149) -> (-44.8339, -40.5925) centre (0, 0) ccw
  arc A43 (-44.8339, -40.5925) -> (-40.5925, -44.8339) centre (-42.7658, -42.7658) ccw
  arc A44 (-40.5925, -44.8339) -> (-36.149, -48.488) centre (0, 0) ccw
  line L33 (-36.149, -48.488) -> (-48.8434, -61.1824)
  line L34 (-48.8434, -61.1824) -> (-61.1824, -48.8434)
  arc A45 (89.6437, 8) -> (82.5418, 35.8727) centre (0, 0) ccw
  line L35 (89.6437, 8) -> (59.9486, 8)
  arc A46 (59.9486, 8) -> (51.3551, 31.945) centre (0, 0) ccw
  line L36 (51.3551, 31.945) -> (64.7179, 45.3079)
  line L37 (64.7179, 45.3079) -> (78.3474, 31.6784)
  line L38 (78.3474, 31.6784) -> (82.5418, 35.8727)
  circle A47 centre (-39.2975, 55.172) radius 1.65
  circle A48 centre (55.172, 39.2975) radius 1.65
  circle A49 centre (64.0816, 48.207) radius 1.65
  line L39 (61.1824, 48.8434) -> (48.488, 36.149)
  arc A50 (48.488, 36.149) -> (44.8339, 40.5925) centre (0, 0) ccw
  arc A51 (44.8339, 40.5925) -> (40.5925, 44.8339) centre (42.7658, 42.7658) ccw
  arc A52 (40.5925, 44.8339) -> (36.149, 48.488) centre (0, 0) ccw
  line L40 (36.149, 48.488) -> (48.8434, 61.1824)
  line L41 (48.8434, 61.1824) -> (61.1824, 48.8434)
  circle A53 centre (48.1818, 92.7295) radius 1.65
  line L42 (45.3079, 64.7179) -> (31.945, 51.3551)
  arc A54 (31.945, 51.3551) -> (8, 59.9486) centre (0, 0) ccw
  line L43 (8, 59.9486) -> (8, 89.6437)
  arc A55 (35.8727, 82.5418) -> (8, 89.6437) centre (0, 0) ccw
  line L44 (35.8727, 82.5418) -> (31.6784, 78.3474)
  line L45 (31.6784, 78.3474) -> (45.3079, 64.7179)
  circle A56 centre (0, 0) radius 57.48
  arc A57 (-8, 89.6437) -> (-35.8727, 82.5418) centre (0, 0) ccw
  line L46 (-8, 89.6437) -> (-8, 59.9486)
  arc A58 (-8, 59.9486) -> (-31.945, 51.3551) centre (0, 0) ccw
  line L47 (-31.945, 51.3551) -> (-45.3079, 64.7179)
  line L48 (-45.3079, 64.7179) -> (-31.6784, 78.3474)
  line L49 (-31.6784, 78.3474) -> (-35.8727, 82.5418)
  line L50 (45.6582, 92.3273) -> (38.1472, 84.8162)
  arc A59 (38.1472, 84.8162) -> (5, 92.8655) centre (0, 0) ccw
  line L51 (5, 92.8655) -> (5, 60.273)
  line L52 (5, 60.273) -> (-5, 60.273)
  line L53 (-5, 60.273) -> (-5, 92.8655)
  arc A60 (-5, 92.8655) -> (-38.1472, 84.8162) centre (0, 0) ccw
  line L54 (-38.1472, 84.8162) -> (-45.6582, 92.3273)
  arc A61 (45.6582, 92.3273) -> (-45.6582, 92.3273) centre (0, 0) ccw
  circle A62 centre (-48.1818, -92.7295) radius 1.65
  circle A63 centre (-55.172, -39.2975) radius 1.65
  circle A64 centre (-64.0816, -48.207) radius 1.65
  line L55 (38.9921, -76.6906) -> (33.3352, -82.3475)
  arc A65 (33.3352, -82.3475) -> (-33.3352, -82.3475) centre (0, -115.48) ccw
  line L56 (-33.3352, -82.3475) -> (-38.9921, -76.6906)
  arc A66 (38.9921, -76.6906) -> (-38.9921, -76.6906) centre (0, -115.48) ccw
  line L57 (38.7495, -78.3474) -> (78.3474, -38.7495)
  line L58 (78.3474, -38.7495) -> (93.5553, -53.9574)
  arc A67 (93.5553, -53.9574) -> (93.5553, 53.9574) centre (0, 0) ccw
  line L59 (93.5553, 53.9574) -> (78.3474, 38.7495)
  line L60 (78.3474, 38.7495) -> (38.7495, 78.3474)
  line L61 (38.7495, 78.3474) -> (53.9574, 93.5553)
  arc A68 (53.9574, 93.5553) -> (-53.9574, 93.5553) centre (0, 0) ccw
  line L62 (-53.9574, 93.5553) -> (-38.7495, 78.3474)
  line L63 (-38.7495, 78.3474) -> (-78.3474, 38.7495)
  line L64 (-78.3474, 38.7495) -> (-93.5553, 53.9574)
  arc A69 (-93.5553, 53.9574) -> (-93.5553, -53.9574) centre (0, 0) ccw
  line L65 (-93.5553, -53.9574) -> (-78.3474, -38.7495)
  line L66 (-78.3474, -38.7495) -> (-38.7495, -78.3474)
  line L67 (-38.7495, -78.3474) -> (-53.9574, -93.5553)
  arc A70 (-53.9574, -93.5553) -> (-42.0574, -99.4745) centre (0, 0) ccw
  arc A71 (42.0574, -99.4745) -> (-42.0574, -99.4745) centre (0, -115.48) ccw
  arc A72 (42.0574, -99.4745) -> (53.9574, -93.5553) centre (0, 0) ccw
  line L68 (53.9574, -93.5553) -> (38.7495, -78.3474)
  circle A73 centre (-48.1818, 92.7295) radius 1.65
  line L69 (88.5718, -41.9027) -> (92.1073, -38.3672)
  line L70 (92.1073, -38.3672) -> (86.8909, -33.1508)
  line L71 (92.1073, -38.3672) -> (94.5642, -40.8241)
  line L72 (92.3273, -45.6582) -> (86.8909, -33.1508)
  line L73 (94.5642, -40.8241) -> (84.8162, -38.1472)
  circle A74 centre (89.6381, -39.4713) radius 1.45
  line L74 (88.5718, 41.9027) -> (92.1073, 38.3672)
  line L75 (92.1073, 38.3672) -> (94.5642, 40.8241)
  line L76 (94.5642, 40.8241) -> (86.8909, 33.1508)
  line L77 (92.3273, 45.6582) -> (86.8909, 33.1508)
  line L78 (84.8162, 38.1472) -> (94.5642, 40.8241)
  circle A75 centre (89.6381, 39.4713) radius 1.45
  line L79 (41.9027, 88.5718) -> (38.3672, 92.1073)
  line L80 (38.3672, 92.1073) -> (40.8241, 94.5642)
  line L81 (40.8241, 94.5642) -> (33.1508, 86.8909)
  line L82 (45.6582, 92.3273) -> (33.1508, 86.8909)
  line L83 (40.8241, 94.5642) -> (38.1472, 84.8162)
  circle A76 centre (39.4713, 89.6381) radius 1.45
  line L84 (-41.9027, 88.5718) -> (-38.3672, 92.1073)
  line L85 (-38.3672, 92.1073) -> (-33.1508, 86.8909)
  line L86 (-33.1508, 86.8909) -> (-40.8241, 94.5642)
  line L87 (-40.8241, 94.5642) -> (-38.1472, 84.8162)
  line L88 (-33.1508, 86.8909) -> (-45.6582, 92.3273)
  circle A77 centre (-39.4713, 89.6381) radius 1.45
  line L89 (-88.5718, -41.9027) -> (-92.1073, -38.3672)
  line L90 (-92.1073, -38.3672) -> (-86.8909, -33.1508)
  line L91 (-86.8909, -33.1508) -> (-94.5642, -40.8241)
  line L92 (-86.8909, -33.1508) -> (-92.3273, -45.6582)
  line L93 (-84.8162, -38.1472) -> (-94.5642, -40.8241)
  circle A78 centre (-89.6381, -39.4713) radius 1.45
  line L94 (-88.5718, 41.9027) -> (-92.1073, 38.3672)
  line L95 (-92.1073, 38.3672) -> (-94.5642, 40.8241)
  line L96 (-94.5642, 40.8241) -> (-86.8909, 33.1508)
  line L97 (-86.8909, 33.1508) -> (-92.3273, 45.6582)
  line L98 (-84.8162, 38.1472) -> (-94.5642, 40.8241)
  circle A79 centre (-89.6381, 39.4713) radius 1.45
  line L99 (-54.2065, -33.8065) -> (-56.6814, -31.3316)
  circle A80 centre (-56.6814, -31.3316) radius 2.5
  line L100 (-56.6814, -31.3316) -> (-53.5193, -28.1695)
  line L101 (-54.2065, -33.8065) -> (-53.7115, -34.3014)
  line L102 (-56.6814, -31.3316) -> (-58.4491, -29.5638)
  line L103 (-58.4491, -29.5638) -> (-54.6959, -25.8106)
  line L104 (-56.6814, -31.3316) -> (-58.4491, -33.0994)
  line L105 (-58.4491, -33.0994) -> (-55.4793, -36.0692)
  circle A81 centre (-56.6814, -31.3316) radius 1.65
  line L106 (-1.75, 0) -> (-22.5, 0)
  line L107 (-58.4491, 29.5638) -> (-54.6959, 25.8106)
  line L108 (-56.6814, 31.3316) -> (-53.5193, 28.1695)
  line L109 (-54.2065, 33.8065) -> (-53.7115, 34.3014)
  line L110 (-54.2065, 33.8065) -> (-56.6814, 31.3316)
  line L111 (-58.4491, 33.0994) -> (-55.4793, 36.0692)
  circle A82 centre (-56.6814, 31.3316) radius 2.5
  circle A83 centre (-56.6814, 31.3316) radius 1.65
  line L112 (-56.6814, 31.3316) -> (-58.4491, 29.5638)
  line L113 (-56.6814, 31.3316) -> (-58.4491, 33.0994)
  line L114 (0, -1.75) -> (0, -22.5)
  line L115 (58.4491, -33.0994) -> (55.4793, -36.0692)
  line L116 (54.2065, -33.8065) -> (56.6814, -31.3316)
  line L117 (54.2065, -33.8065) -> (53.7115, -34.3014)
  circle A84 centre (56.6814, -31.3316) radius 2.5
  circle A85 centre (56.6814, -31.3316) radius 1.65
  line L118 (56.6814, -31.3316) -> (58.4491, -33.0994)
  line L119 (56.6814, -31.3316) -> (58.4491, -29.5638)
  line L120 (56.6814, -31.3316) -> (53.5193, -28.1695)
  line L121 (58.4491, -29.5638) -> (54.6959, -25.8106)
  line L122 (58.4491, 29.5638) -> (54.6959, 25.8106)
  line L123 (56.6814, 31.3316) -> (53.5193, 28.1695)
  circle A86 centre (56.6814, 31.3316) radius 2.5
  circle A87 centre (56.6814, 31.3316) radius 1.65
  line L124 (56.6814, 31.3316) -> (58.4491, 33.0994)
  line L125 (56.6814, 31.3316) -> (58.4491, 29.5638)
  line L126 (54.2065, 33.8065) -> (53.7115, 34.3014)
  line L127 (54.2065, 33.8065) -> (56.6814, 31.3316)
  line L128 (58.4491, 33.0994) -> (55.4793, 36.0692)
  line L129 (-29.5638, -58.4491) -> (-25.8106, -54.6959)
  circle A88 centre (-31.3316, -56.6814) radius 2.5
  circle A89 centre (-31.3316, -56.6814) radius 1.65
  line L130 (-31.3316, -56.6814) -> (-28.1695, -53.5193)
  line L131 (-31.3316, -56.6814) -> (-33.0994, -58.4491)
  line L132 (-31.3316, -56.6814) -> (-29.5638, -58.4491)
  line L133 (-33.8065, -54.2065) -> (-31.3316, -56.6814)
  line L134 (-33.0994, -58.4491) -> (-36.0692, -55.4793)
  line L135 (-33.8065, -54.2065) -> (-34.3014, -53.7115)
  line L136 (33.8065, -54.2065) -> (31.3316, -56.6814)
  line L137 (33.8065, -54.2065) -> (34.3014, -53.7115)
  line L138 (33.0994, -58.4491) -> (36.0692, -55.4793)
  circle A90 centre (31.3316, -56.6814) radius 2.5
  circle A91 centre (31.3316, -56.6814) radius 1.65
  line L139 (31.3316, -56.6814) -> (33.0994, -58.4491)
  line L140 (31.3316, -56.6814) -> (29.5638, -58.4491)
  line L141 (31.3316, -56.6814) -> (28.1695, -53.5193)
  line L142 (29.5638, -58.4491) -> (25.8106, -54.6959)
  line L143 (58.4491, -29.5638) -> (54.6959, -25.8106)
  circle A92 centre (56.6814, -31.3316) radius 2.5
  circle A93 centre (56.6814, -31.3316) radius 1.65
  line L144 (56.6814, -31.3316) -> (53.5193, -28.1695)
  line L145 (56.6814, -31.3316) -> (58.4491, -33.0994)
  line L146 (56.6814, -31.3316) -> (58.4491, -29.5638)
  line L147 (54.2065, -33.8065) -> (56.6814, -31.3316)
  line L148 (58.4491, -33.0994) -> (55.4793, -36.0692)
  line L149 (54.2065, -33.8065) -> (53.7115, -34.3014)
  line L150 (54.2065, 33.8065) -> (56.6814, 31.3316)
  line L151 (54.2065, 33.8065) -> (53.7115, 34.3014)
  line L152 (58.4491, 33.0994) -> (55.4793, 36.0692)
  circle A94 centre (56.6814, 31.3316) radius 2.5
  circle A95 centre (56.6814, 31.3316) radius 1.65
  line L153 (56.6814, 31.3316) -> (58.4491, 33.0994)
  line L154 (56.6814, 31.3316) -> (58.4491, 29.5638)
  line L155 (56.6814, 31.3316) -> (53.5193, 28.1695)
  line L156 (58.4491, 29.5638) -> (54.6959, 25.8106)
  line L157 (29.5638, 58.4491) -> (25.8106, 54.6959)
  circle A96 centre (31.3316, 56.6814) radius 2.5
  circle A97 centre (31.3316, 56.6814) radius 1.65
  line L158 (31.3316, 56.6814) -> (28.1695, 53.5193)
  line L159 (31.3316, 56.6814) -> (33.0994, 58.4491)
  line L160 (31.3316, 56.6814) -> (29.5638, 58.4491)
  line L161 (33.8065, 54.2065) -> (31.3316, 56.6814)
  line L162 (33.0994, 58.4491) -> (36.0692, 55.4793)
  line L163 (33.8065, 54.2065) -> (34.3014, 53.7115)
  line L164 (-33.8065, 54.2065) -> (-31.3316, 56.6814)
  line L165 (-33.8065, 54.2065) -> (-34.3014, 53.7115)
  line L166 (-33.0994, 58.4491) -> (-36.0692, 55.4793)
  circle A98 centre (-31.3316, 56.6814) radius 2.5
  circle A99 centre (-31.3316, 56.6814) radius 1.65
  line L167 (-31.3316, 56.6814) -> (-33.0994, 58.4491)
  line L168 (-31.3316, 56.6814) -> (-29.5638, 58.4491)
  line L169 (-31.3316, 56.6814) -> (-28.1695, 53.5193)
  line L170 (-29.5638, 58.4491) -> (-25.8106, 54.6959)
  dimension "d78" = 5
  dimension "d79" = 2.9
  dimension "d80" = 5
  dimension "d81" = 2.9
  dimension "d82" = 5
  dimension "d83" = 2.9
  dimension "d84" = 5
  dimension "d85" = 2.9
  dimension "d86" = 5
  dimension "d87" = 2.9
  dimension "d88" = 5
  dimension "d89" = 2.9
  dimension "d105" = 3.5
  dimension "d106" = 5
  dimension "d107" = 3.3
  dimension "d109" = 360
  constraint midpoint L24 L69.start
  constraint perpendicular L24 L69
  constraint coincident A34 L70.end
  constraint perpendicular L69 L70
  constraint coincident A33 L71.end
  constraint perpendicular L69 L71
  constraint coincident A33.start L24.start
  constraint coincident L24.end A34.start
  constraint coincident L72 A74.centre
  constraint coincident L73 A74.centre
  constraint midpoint L28 L74.start
  constraint perpendicular L28 L74
  constraint coincident A33 L75.end
  constraint perpendicular L74 L75
  constraint coincident A35 L76.end
  constraint parallel L75 L76
  constraint coincident A33.end L28.end
  constraint coincident A35.end L28.start
  constraint coincident L77 A75.centre
  constraint coincident L78 A75.centre
  constraint midpoint L50 L79.start
  constraint perpendicular L50 L79
  constraint coincident A61 L80.end
  constraint perpendicular L79 L80
  constraint coincident A59 L81.end
  constraint parallel L80 L81
  constraint coincident L50.start A61.start
  constraint coincident L50.end A59.start
  constraint coincident L83 A76.centre
  constraint coincident L82 A76.centre
  constraint midpoint L54 L84.start
  constraint perpendicular L54 L84
  constraint coincident A60 L85.end
  constraint perpendicular L84 L85
  constraint coincident A61 L86.end
  constraint parallel L85 L86
  constraint coincident A60.end L54.start
  constraint coincident L54.end A61.end
  constraint coincident L88 A77.centre
  constraint coincident L87 A77.centre
  constraint midpoint L19 L89.start
  constraint perpendicular L19 L89
  constraint coincident A22 L90.end
  constraint perpendicular L89 L90
  constraint coincident A20 L91.end
  constraint parallel L90 L91
  constraint coincident A20.end L19.end
  constraint coincident A22.end L19.start
  constraint coincident L93 A78.centre
  constraint coincident L92 A78.centre
  constraint midpoint L15 L94.start
  constraint perpendicular L15 L94
  constraint coincident A20 L95.end
  constraint perpendicular L94 L95
  constraint coincident A21 L96.end
  constraint parallel L95 L96
  constraint coincident A20.start L15.start
  constraint coincident L15.end A21.start
  constraint coincident L97 A79.centre
  constraint coincident L98 A79.centre
  constraint coincident L99.end A80.centre
  constraint coincident A11 L100.end
  constraint perpendicular L99 L100
  constraint coincident L10 L101.end
  constraint perpendicular L10 L101
  constraint coincident A80 L102.end
  constraint perpendicular L100 L102
  constraint coincident A11 L103.end
  constraint tangent A80 L103
  constraint coincident A80 L104.end
  constraint perpendicular L99 L104
  constraint coincident L10 L105.end
  constraint tangent A80 L105
  constraint perpendicular L10 L105
  constraint concentric A80 A81
  constraint symmetric L99.start L106 L109.start
  constraint symmetric L99.end L106 L108.start
  constraint symmetric A80 L106 A82
  constraint symmetric L100.end L106 L108.end
  constraint symmetric L101.end L106 L109.end
  constraint symmetric L102.end L106 L107.start
  constraint symmetric L103.end L106 L107.end
  constraint symmetric L104.end L106 L111.start
  constraint symmetric L105.end L106 L111.end
  constraint symmetric A81 L106 A83
  constraint symmetric L99.start L114 L116.start
  constraint symmetric L99.end L114 L116.end
  constraint symmetric A80 L114 A84
  constraint symmetric L100.end L114 L120.end
  constraint symmetric L101.end L114 L117.end
  constraint symmetric L102.end L114 L119.end
  constraint symmetric L103.end L114 L121.end
  constraint symmetric L104.end L114 L115.start
  constraint symmetric L105.end L114 L115.end
  constraint symmetric A81 L114 A85
  constraint symmetric L107.start L114 L122.start
  constraint symmetric L107.end L114 L122.end
  constraint symmetric L108.start L114 L123.start
  constraint symmetric L108.end L114 L123.end
  constraint symmetric L109.start L114 L126.start
  constraint symmetric L109.end L114 L126.end
  constraint symmetric L111.start L114 L124.end
  constraint symmetric L111.end L114 L128.end
  constraint symmetric A82 L114 A86
  constraint symmetric A83 L114 A87
  measures "d78" distance of L69.start L69.end
  measures "d79" diameter of A74
  measures "d80" distance of L74.start L74.end
  measures "d81" diameter of A75
  measures "d82" distance of L79.start L79.end
  measures "d83" diameter of A76
  measures "d84" distance of L84.start L84.end
  measures "d85" diameter of A77
  measures "d86" distance of L89.start L89.end
  measures "d87" diameter of A78
  measures "d88" distance of L94.start L94.end
  measures "d89" diameter of A79
  measures "d105" distance of L99.start L99.end
  measures "d106" diameter of A80
  measures "d107" diameter of A81